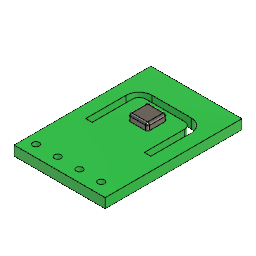
Smart-FrameV2 v15 (Autodesk Fusion 360 archive; units mm, degrees)
design "BME680"
Autodesk Fusion 360 part; units mm, degrees
sketch "Sketch1" plane through (0, 0, 0) normal (0, 0, 1) x (1, 0, 0)
  line L0 (0, 0) -> (14, 0)
  line L1 (14, 0) -> (14, 21)
  line L2 (14, 21) -> (0, 21)
  line L3 (0, 21) -> (0, 0)
  line L4 (2, 9) -> (2, 15.2)
  line L5 (4, 17.2) -> (10, 17.2)
  line L6 (12, 15.2) -> (12, 9)
  line L7 (12, 9) -> (11, 9)
  line L8 (11, 9) -> (11, 15.2)
  line L9 (10, 16.2) -> (4, 16.2)
  line L10 (3, 15.2) -> (3, 9)
  line L11 (3, 9) -> (2, 9)
  line L12 (7, 19.5138) -> (7, 1.832) construction
  arc A0 (4, 16.2) -> (3, 15.2) centre (4, 15.2) ccw
  arc A1 (11, 15.2) -> (10, 16.2) centre (10, 15.2) ccw
  arc A2 (4, 17.2) -> (2, 15.2) centre (4, 15.2) ccw
  arc A3 (12, 15.2) -> (10, 17.2) centre (10, 15.2) ccw
  dimension "d1" = 14
  dimension "d2" = 21
  dimension "d5" = 1
  dimension "d6" = 1
  dimension "d7" = 2
  dimension "d8" = 1
  dimension "d9" = 1
  dimension "d10" = 2
  dimension "d11" = 3.8
  dimension "d12" = 9
  dimension "d13" = 2
  constraint horizontal L0
  constraint vertical L1
  constraint horizontal L2
  constraint vertical L3
  constraint coincident L0.start L3.end
  constraint vertical L4
  constraint perpendicular L4 L5
  constraint perpendicular L5 L6
  constraint perpendicular L6 L7
  constraint perpendicular L7 L8
  constraint perpendicular L8 L9
  constraint perpendicular L9 L10
  constraint horizontal L11
  constraint equal L7 L11
  constraint vertical L12
  constraint symmetric L8 L10 L12
  constraint collinear L7 L11
  constraint tangent L9 A0
  constraint tangent L10 A0
  constraint tangent L9 A1
  constraint tangent L8 A1
  constraint tangent L5 A2
  constraint tangent L4 A2
  constraint tangent L6 A3
  constraint tangent L5 A3
  constraint equal A2 A3
  measures "d1" distance of L0.start L0.end
  measures "d2" distance of L0.start L2.end
  measures "d5" distance of L4.start L10.end
  measures "d6" distance of L5 L9
  measures "d7" distance of L3 L4
  measures "d8" radius of A0
  measures "d9" radius of A1
  measures "d10" radius of A2
  measures "d11" distance of L2 L5
  measures "d12" distance of L0 L11
  measures "d13" distance of L1 L6
extrude "Extrude1" add sketch "Sketch1" along normal blind 1.5
hole "Hole1" at (1.6, 1.8, 1.5) direction (0, 0, -1) diameter 1 depth 5 tip angle 118
pattern_linear "R-Pattern1" count 4 spacing 3.3333 along (1, 0, 0) of "Hole1"
sketch "Sketch3" plane through (0, 0, 1.5) normal (0, 0, 1) x (-1, 0, 0)
  circle A0 centre (-11.6, -1.8) radius 0.5
  circle A1 centre (-8.2667, -1.8) radius 0.5
  circle A2 centre (-4.9333, -1.8) radius 0.5
  circle A3 centre (-1.6, -1.8) radius 0.5
  line L0 (-12, -15.2) -> (-12, -9)
  line L1 (-12, -9) -> (-11, -9)
  line L2 (-11, -9) -> (-11, -15.2)
  arc A4 (-11, -15.2) -> (-10, -16.2) centre (-10, -15.2) ccw
  line L3 (-10, -16.2) -> (-4, -16.2)
  arc A5 (-4, -16.2) -> (-3, -15.2) centre (-4, -15.2) ccw
  line L4 (-3, -15.2) -> (-3, -9)
  line L5 (-3, -9) -> (-2, -9)
  line L6 (-2, -9) -> (-2, -15.2)
  arc A6 (-4, -17.2) -> (-2, -15.2) centre (-4, -15.2) ccw
  line L7 (-4, -17.2) -> (-10, -17.2)
  arc A7 (-12, -15.2) -> (-10, -17.2) centre (-10, -15.2) ccw
  line L8 (0, -21) -> (0, 0)
  line L9 (0, 0) -> (-14, 0)
  line L10 (-14, 0) -> (-14, -21)
  line L11 (-14, -21) -> (0, -21)
  line L12 (-5.5, -15) -> (-8.5, -15)
  line L13 (-8.5, -15) -> (-8.5, -12)
  line L14 (-8.5, -12) -> (-5.5, -12)
  line L15 (-5.5, -12) -> (-5.5, -15)
  dimension "d23" = 3
  dimension "d24" = 3
  dimension "d25" = 6
  dimension "d26" = 5.5
  constraint horizontal L12
  constraint vertical L13
  constraint horizontal L14
  constraint vertical L15
  measures "d23" distance of L12.start L12.end
  measures "d24" distance of L12.end L13.end
  measures "d25" distance of L11 L12
  measures "d26" distance of L8 L15
extrude "Extrude2" add sketch "Sketch3" along normal blind 1 contours L12 L13 L14 L15
fillet "Fillet1" radius 0.3 8 edges at (5.5, 15, 2) (8.5, 15, 2) (8.5, 12, 2) (5.5, 12, 2) (7, 12, 2.5) (5.5, 13.5, 2.5) (8.5, 13.5, 2.5) (7, 15, 2.5)
ref_plane "WorkPlane1" through (7, 13.5, 2) normal (0, 1, 0) x (-1, 0, 0)

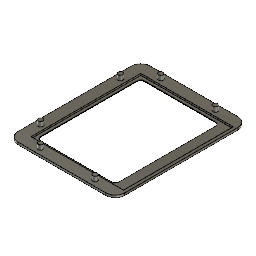
design "FrameF"
Autodesk Fusion 360 part; units mm, degrees
sketch "Sketch1" plane through (0, 0, 0) normal (0, 0, 1) x (1, 0, 0)
  line L0 (-4.3711, 0) -> (69.6289, 0)
  line L1 (77.6289, 8) -> (77.6289, 103.4)
  line L2 (69.6289, 111.4) -> (-4.3711, 111.4)
  line L3 (-12.3711, 103.4) -> (-12.3711, 8)
  arc A0 (-4.3711, 111.4) -> (-12.3711, 103.4) centre (-4.3711, 103.4) ccw
  arc A1 (77.6289, 103.4) -> (69.6289, 111.4) centre (69.6289, 103.4) ccw
  arc A2 (69.6289, 0) -> (77.6289, 8) centre (69.6289, 8) ccw
  arc A3 (-12.3711, 8) -> (-4.3711, 0) centre (-4.3711, 8) ccw
  line L4 (-0.3711, 12) -> (65.6289, 12)
  line L5 (65.6289, 12) -> (65.6289, 99.4)
  line L6 (65.6289, 99.4) -> (-0.3711, 99.4)
  line L7 (-0.3711, 99.4) -> (-0.3711, 12)
  dimension "d1" = 8
  dimension "d2" = 8
  dimension "d3" = 90
  dimension "d4" = 111.4
  dimension "d5" = 12
  dimension "d6" = 12
  dimension "d7" = 12
  dimension "d8" = 12
  constraint horizontal L0
  constraint vertical L1
  constraint horizontal L2
  constraint vertical L3
  constraint tangent L2 A0
  constraint tangent L3 A0
  constraint tangent L2 A1
  constraint tangent L1 A1
  constraint tangent L1 A2
  constraint tangent L0 A2
  constraint equal A1 A2
  constraint tangent L0 A3
  constraint tangent L3 A3
  constraint equal A1 A3
  constraint horizontal L4
  constraint vertical L5
  constraint horizontal L6
  constraint vertical L7
  measures "d1" radius of A0
  measures "d2" radius of A1
  measures "d3" distance of L1 L3
  measures "d4" distance of L0 L2
  measures "d5" distance of L3 L7
  measures "d6" distance of L0 L4
  measures "d7" distance of L1 L5
  measures "d8" distance of L2 L6
extrude "Extrude1" add sketch "Sketch1" along normal blind 2
fillet "Fillet2" radius 3 4 edges at (65.6289, 12, 1) (-0.3711, 12, 1) (-0.3711, 99.4, 1) (65.6289, 99.4, 1)
chamfer "Chamfer2" [suppressed]
sketch "Sketch2" plane through (0, 0, 2) normal (0, 0, 1) x (-1, 0, 0)
  line L0 (0.3711, -15) -> (0.3711, -96.4)
  line L1 (-2.6289, -99.4) -> (-62.6289, -99.4)
  line L2 (-65.6289, -96.4) -> (-65.6289, -15)
  line L3 (-62.6289, -12) -> (-2.6289, -12)
  arc A0 (12.3711, -8) -> (4.3711, 0) centre (4.3711, -8) ccw
  line L4 (4.3711, 0) -> (-69.6289, 0)
  arc A1 (-69.6289, 0) -> (-77.6289, -8) centre (-69.6289, -8) ccw
  line L5 (-77.6289, -8) -> (-77.6289, -103.4)
  arc A2 (-77.6289, -103.4) -> (-69.6289, -111.4) centre (-69.6289, -103.4) ccw
  line L6 (-69.6289, -111.4) -> (4.3711, -111.4)
  arc A3 (4.3711, -111.4) -> (12.3711, -103.4) centre (4.3711, -103.4) ccw
  line L7 (12.3711, -103.4) -> (12.3711, -8)
  line L8 (2.8711, -101.9) -> (-75.1289, -101.9)
  line L9 (-75.1289, -101.9) -> (-75.1289, -9.5)
  line L10 (-75.1289, -9.5) -> (2.8711, -9.5)
  line L11 (2.8711, -9.5) -> (2.8711, -101.9)
  arc A4 (-2.6289, -99.4) -> (0.3711, -96.4) centre (-2.6289, -96.4) ccw
  arc A5 (-65.6289, -96.4) -> (-62.6289, -99.4) centre (-62.6289, -96.4) ccw
  arc A6 (-62.6289, -12) -> (-65.6289, -15) centre (-62.6289, -15) ccw
  arc A7 (0.3711, -15) -> (-2.6289, -12) centre (-2.6289, -15) ccw
  dimension "d15" = 2.5
  dimension "d16" = 2.5
  dimension "d17" = 2.5
  dimension "d64" = 78
  constraint horizontal L8
  constraint vertical L9
  constraint horizontal L10
  constraint vertical L11
  measures "d15" distance of L0 L11
  measures "d16" distance of L1 L8
  measures "d17" distance of L3 L10
  measures "d64" distance of L9 L11
extrude "Extrude2" cut sketch "Sketch2" against normal blind 1.4 contours L8 L9 L10 L11
sketch "Sketch4" plane through (0, 0, 2) normal (0, 0, 1) x (-1, 0, 0)
  line L0 (-75.1289, -101.9) -> (-75.1289, -9.5)
  line L1 (-75.1289, -9.5) -> (2.8711, -9.5)
  line L2 (2.8711, -9.5) -> (2.8711, -101.9)
  line L3 (2.8711, -101.9) -> (-75.1289, -101.9)
  arc A0 (12.3711, -8) -> (4.3711, 0) centre (4.3711, -8) ccw
  line L4 (4.3711, 0) -> (-69.6289, 0)
  arc A1 (-69.6289, 0) -> (-77.6289, -8) centre (-69.6289, -8) ccw
  line L5 (-77.6289, -8) -> (-77.6289, -103.4)
  arc A2 (-77.6289, -103.4) -> (-69.6289, -111.4) centre (-69.6289, -103.4) ccw
  line L6 (-69.6289, -111.4) -> (4.3711, -111.4)
  arc A3 (4.3711, -111.4) -> (12.3711, -103.4) centre (4.3711, -103.4) ccw
  line L7 (12.3711, -103.4) -> (12.3711, -8)
  line L8 (7.3711, -106.4) -> (-71.5219, -106.4) construction
  line L9 (-71.5219, -106.4) -> (-71.5219, -5) construction
  line L10 (-71.5219, -5) -> (7.3711, -5) construction
  line L11 (7.3711, -5) -> (7.3711, -106.4) construction
  circle A4 centre (-9.6289, -106.4) radius 2
  circle A5 centre (-55.6289, -106.4) radius 2
  circle A6 centre (7.3711, -89.4) radius 2
  circle A7 centre (7.3711, -22) radius 2
  circle A8 centre (-9.6289, -5) radius 2
  circle A9 centre (-55.6289, -5) radius 2
  dimension "d46" = 5
  dimension "d47" = 5
  dimension "d48" = 5
  dimension "d49" = 4
  dimension "d50" = 4
  dimension "d51" = 4
  dimension "d52" = 4
  dimension "d53" = 4
  dimension "d54" = 4
  dimension "d55" = 22
  dimension "d56" = 22
  dimension "d57" = 22
  dimension "d58" = 22
  dimension "d59" = 22
  dimension "d60" = 22
  constraint horizontal L8
  constraint vertical L9
  constraint horizontal L10
  constraint vertical L11
  constraint coincident L8 A4.centre
  constraint coincident L8 A5.centre
  constraint coincident L11 A6.centre
  constraint coincident L11 A7.centre
  constraint coincident L10 A8.centre
  constraint coincident L10 A9.centre
  measures "d46" distance of L6 L8
  measures "d47" distance of L7 L11
  measures "d48" distance of L4 L10
  measures "d49" diameter of A4
  measures "d50" diameter of A5
  measures "d51" diameter of A6
  measures "d52" diameter of A7
  measures "d53" diameter of A8
  measures "d54" diameter of A9
  measures "d55" distance of L7 A4.centre
  measures "d56" distance of L5 A5.centre
  measures "d57" distance of L6 A6.centre
  measures "d58" distance of L4 A7.centre
  measures "d59" distance of L7 A8.centre
  measures "d60" distance of L5 A9.centre
extrude "Extrude4" add sketch "Sketch4" along normal blind 4 contours A4 | A5 | A6 | A7 | A8 | A9
